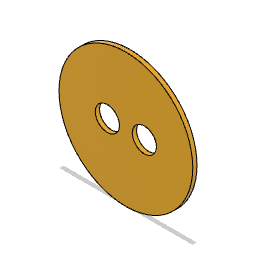
Lid (Autodesk Fusion 360 design; units mm, degrees)
Autodesk Fusion 360 part; units mm, degrees
sketch "Sketch1" plane through (0, 0, 0) normal (0, 0, 1) x (1, 0, 0)
  circle A0 centre (0, 0) radius 47
  dimension "d1" = 94
  constraint coincident A0.centre origin
  measures "d1" diameter of A0
extrude "Extrude1" add sketch "Sketch1" along normal blind 3
sketch "Sketch5" plane through (0, 0, 3) normal (0, 0, 1) x (1, 0, 0)
  circle A0 centre (0, 0) radius 47
  circle A1 through (21.5, 0, -3) (8.75, 7.3612, -3) (8.75, -7.3612, -3)
  dimension "d4" = 17
extrude "Extrude2" cut sketch "Sketch5" along normal blind 3 contours A1 in plane through (0, 0, 0) normal (0, 0, 1)
sketch "Sketch6" plane through (0, 0, 3) normal (0, 0, 1) x (1, 0, 0)
  circle A0 centre (13, 0) radius 8.5
  circle A1 centre (0, 0) radius 47
  circle A2 through (-4.5, 0, -3) (-17.25, 7.3612, -3) (-17.25, -7.3612, -3)
  dimension "d7" = 17
extrude "Extrude3" cut sketch "Sketch6" along normal blind 3 contours A2 in plane through (0, 0, 0) normal (0, 0, 1)
move_body "Move1" bodies 1 to x (1, 0, 0) y (0, 1, 0) z (0, 0, 1) at (0, 0, 73)
